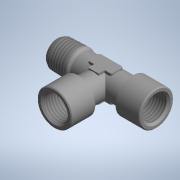
# Autodesk Inventor part: 8030247 NPFC-T-2G14-R14-FMF
Saved by Autodesk Inventor 2021 (Build 250183000, 183)
## iProperties
Part Number: 8030247 NPFC-T-2G14-R14-FMF
Material: Generic
Catalog Web Link: www.cadenas.de
Description: NPFC-T-T-fitting
Vendor: FESTO
Document SubType Name: Modeling
Designer: partserver
Manufacturer: FESTO
Mass: 44.4 g
Surface Area: 51.9093 cm^2
Volume: 5.63168 cm^3
Density: 7.88398 g/cm^3
Appearance: PSOLRGB-175-175-175
Category: PARTsolutions
Company: FESTO
PSOL_IDENT_0: {$CADENAS_DATA\23d-libs\festo\parts\n\npfc\npfc_t.prj},195 {VTYP=3D},{NB=8030247 NPFC-T-2G14-R14-FMF
PSOL_IDENT_1: },{LINA=8030247 NPFC-T-2G14-R14-FMF},{NN=NPFC-T},{DATE=17.05.2021 10:41:53},{GEOMDATE=19.12.2018 13:
PSOL_IDENT_2: 12:53},{VERSION=},{LINEID=460},{WBVAR=},{WBNUMERIC=}  {NB=8030247 NPFC-T-2G14-R14-FMF},{LINA=8030247
PSOL_IDENT_3: NPFC-T-2G14-R14-FMF},{KT=DUMMY},{TNR=8030247},{TYP=NPFC-T-2G14-R14-FMF},{VERS=8},{D=0.0},{D1=8.000}
PSOL_IDENT_4: ,{D2=8.0},{D4=12.000},{T=0},{TC=0.000},{T1=G1/4},{T1C=13.157},{T2=R1/4},{T2C=13.157},{A=0.0},{A1=9.5
PSOL_IDENT_5: },{A2=11.0},{A3=0.000},{B=47.50},{E=32.75},{L=23.0},{P=16.5},{SW=13},{CNSMASSEXACT=0.0444},{VERS2=2}
NB: 8030247 NPFC-T-2G14-R14-FMF
NN: NPFC-T
NT: T-fitting
NBSYN: $TNR. $TYP.
LINA: 8030247 NPFC-T-2G14-R14-FMF
CATALOG: Festo
TNR: 8030247
TYP: NPFC-T-2G14-R14-FMF
D: 0
D1: 8
D2: 8
D4: 12
T: 0
T1: G1/4
T2: R1/4
A: 0
A1: 9.5
A2: 11
A3: 0
B: 47.5
E: 32.75
L: 23
P: 16.5
SW: 13
CNSMASSEXACT: 0.0444
SUPPLIER: FESTO
ARTICLENO: 8030247 NPFC-T-2G14-R14-FMF
BOMINFO: 8030247 NPFC-T-2G14-R14-FMF
CREATOR: CADENAS GmbH
Title: 8030247 NPFC-T-2G14-R14-FMF
Author: Cadenas PARTsolutions
Comments: T-fitting
Autodesk Inventor part; units mm, degrees
sketch "Sketch_10" plane through (0, 0, 0) normal (0, 0, 1) x (1, 0, 0)
  line L0 (-5.775, 1.8563) -> (-5.775, -1.8563)
  arc A0 (-5.775, -1.8563) -> (-4.7438, -2.8875) centre (-4.7437, -1.8562) ccw
  line L1 (-4.7438, -2.8875) -> (-2.8188, -2.8875)
  arc A1 (-2.475, -3.2313) -> (-2.8188, -2.8875) centre (-2.8187, -3.2312) ccw
  line L2 (-2.475, -3.2313) -> (-2.475, -5.4313)
  arc A2 (-2.475, -5.4313) -> (-2.1313, -5.775) centre (-2.1313, -5.4313) ccw
  line L3 (-2.1313, -5.775) -> (2.1313, -5.775)
  arc A3 (2.1313, -5.775) -> (2.475, -5.4313) centre (2.1313, -5.4313) ccw
  line L4 (2.475, -5.4313) -> (2.475, -3.2313)
  arc A4 (2.8188, -2.8875) -> (2.475, -3.2313) centre (2.8187, -3.2312) ccw
  line L5 (2.8188, -2.8875) -> (4.7438, -2.8875)
  arc A5 (4.7438, -2.8875) -> (5.775, -1.8563) centre (4.7437, -1.8562) ccw
  line L6 (5.775, -1.8563) -> (5.775, 1.8563)
  arc A6 (5.775, 1.8563) -> (4.7438, 2.8875) centre (4.7437, 1.8562) ccw
  line L7 (4.7438, 2.8875) -> (-4.7438, 2.8875)
  arc A7 (-4.7438, 2.8875) -> (-5.775, 1.8563) centre (-4.7437, 1.8562) ccw
  constraints: 16 end point, 16 point on circle, 8 centre point
extrude "Extrusion1" add sketch "Sketch_10" along normal mid plane 13
sketch "Sketch_25" plane through (0, 0, 0) normal (0, 0, 1) x (1, 0, 0)
  line L0 (-0.75, 0) -> (-24.5, 0)
  line L1 (-24.5, 0) -> (-24.5, 7.8375)
  line L2 (-24.5, 7.8375) -> (-24.0875, 8.25)
  line L3 (-24.0875, 8.25) -> (-13.1, 8.25)
  line L4 (-13.1, 8.25) -> (-11.801, 6)
  line L5 (-11.801, 6) -> (0, 6)
  line L6 (0, 6) -> (0, 0)
  line L7 (0, 0) -> (-24.5, 0)
  constraints: 16 end point
revolve "Revolution1" add sketch "Sketch_25" angle 360 about axis through (-0.75, 0, 0) along (1, 0, 0)
sketch "Sketch_26" plane through (0, 0, 0) normal (0, 0, 1) x (1, 0, 0)
  line L0 (0, -24.5) -> (0, -0.75)
  line L1 (0, 0) -> (6, 0)
  line L2 (6, 0) -> (6, -11.801)
  line L3 (6, -11.801) -> (8.25, -13.1)
  line L4 (8.25, -13.1) -> (8.25, -24.0875)
  line L5 (8.25, -24.0875) -> (7.8375, -24.5)
  line L6 (7.8375, -24.5) -> (0, -24.5)
  line L7 (0, -24.5) -> (0, 0)
  constraints: 16 end point
revolve "Revolution2" add sketch "Sketch_26" angle 360 about axis through (0, -24.5, 0) along (0, -1, 0)
sketch "Sketch_31" plane through (0, 0, 0) normal (0, 0, 1) x (1, 0, 0)
  line L0 (0, 0) -> (23, 0)
  line L1 (23, 0) -> (23, -5.5352)
  line L2 (23, -5.5352) -> (21.4326, -6.4401)
  line L3 (21.4326, -6.4401) -> (12, -6.7346)
  line L4 (12, -6.7346) -> (10.9, -6)
  line L5 (10.9, -6) -> (0, -6)
  line L6 (0, -6) -> (0, 0)
  line L7 (0, 0) -> (23, 0)
  constraints: 16 end point
revolve "Revolution3" add sketch "Sketch_31" angle 360 about axis through (0, 0, 0) along (-1, 0, 0)
thread "Thread1" size "R 1/4" standard "ISO Taper" length 8.4367
sketch "Sketch5" plane through (23, 0, 0) normal (1, 0, 0) x (0, 0, -1)
  point P0 (0, 0)
hole "Hole1" at (23, 0, 0) direction (-1, 0, 0) diameter 8 depth 23 countersink diameter 9.6 countersink angle 90
sketch "Sketch_33" plane through (0, 0, 0) normal (0, 0, 1) x (1, 0, 0)
  line L0 (0, -24.5) -> (0, -0.75)
  line L1 (0, 0) -> (4, 0)
  line L2 (4, 0) -> (4, -12.3689)
  line L3 (4, -12.3689) -> (5.7225, -13.575)
  line L4 (5.7225, -13.575) -> (5.7225, -23.644)
  line L5 (5.7225, -23.644) -> (6.5785, -24.5)
  line L6 (6.5785, -24.5) -> (0, -24.5)
  line L7 (0, -24.5) -> (0, 0)
  constraints: 16 end point
revolve "Revolution4" cut sketch "Sketch_33" angle 360 about axis through (0, -24.5, 0) along (0, -1, 0)
thread "Thread2" size "G13.157x1.337" designation "G 1/4" standard "ISO Pipe Threads" length 8.644
sketch "Sketch_32" plane through (0, 0, 0) normal (0, 0, 1) x (1, 0, 0)
  line L0 (-24.5, 0) -> (-0.75, 0)
  line L1 (0, 0) -> (0, -4)
  line L2 (0, -4) -> (-12.3689, -4)
  line L3 (-12.3689, -4) -> (-13.575, -5.7225)
  line L4 (-13.575, -5.7225) -> (-23.644, -5.7225)
  line L5 (-23.644, -5.7225) -> (-24.5, -6.5785)
  line L6 (-24.5, -6.5785) -> (-24.5, 0)
  line L7 (-24.5, 0) -> (0, 0)
  constraints: 16 end point
revolve "Revolution5" cut sketch "Sketch_32" angle 360 about axis through (-24.5, 0, 0) along (-1, 0, 0)
thread "Thread3" size "G13.157x1.337" designation "G 1/4" standard "ISO Pipe Threads" length 8.644
ref_plane "IPF_XY" through (12.75, 0, 0) normal (-1, 0, 0) x (0, 0, -1)
ref_plane "IPF_YZ" through (12.75, 0, 0) normal (0, 0, -1) x (0, -1, 0)
ref_plane "IPF_ZX" through (12.75, 0, 0) normal (0, -1, 0) x (-1, 0, 0)
ref_plane "IPM1_XY" through (-24.5, 0, 0) normal (1, 0, 0) x (0, 0, -1)
ref_plane "IPM1_YZ" through (-24.5, 0, 0) normal (0, 0, -1) x (0, 1, 0)
ref_plane "IPM1_ZX" through (-24.5, 0, 0) normal (0, 1, 0) x (1, 0, 0)
ref_plane "IPM2_XY" through (0, -24.5, 0) normal (0, 1, 0) x (1, 0, 0)
ref_plane "IPM2_YZ" through (0, -24.5, 0) normal (1, 0, 0) x (0, 0, -1)
ref_plane "IPM2_ZX" through (0, -24.5, 0) normal (0, 0, -1) x (0, 1, 0)
body "Solid1"
